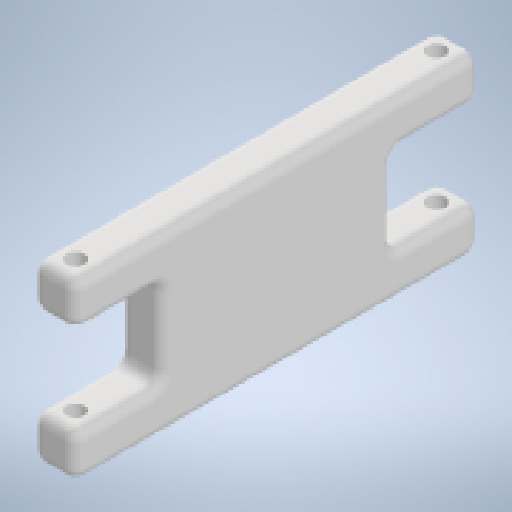
# Autodesk Inventor part: swing pusher
Saved by Autodesk Inventor 2023 (Build 270158000, 158)
## iProperties
Created: 2023-01-25
Part Number: swing pusher
Material: Generic
Document SubType Name: Modeling
Designer: Gabriel - T3 CAD
Density: 1 g/cm^3
Appearance: Default
Mass: 40.324 g
Surface Area: 106.324 cm^2
Volume: 40.324 cm^3
Author: Gabriel - T3 CAD
Autodesk Inventor part; units mm, degrees
ref_plane "YZ Plane" through (0, 0, 0) normal (1, 0, 0) x (0, 1, 0)
ref_plane "XZ Plane" through (0, 0, 0) normal (0, 1, 0) x (-1, 0, 0)
ref_plane "XY Plane" through (0, 0, 0) normal (0, 0, 1) x (1, 0, 0)
sketch "Sketch1" plane through (0, 0, 0) normal (0, 1, 0) x (-1, 0, 0)
  line L0 (0, 0) -> (12.7, 0)
  line L1 (12.7, 0) -> (12.7, 109.3393)
  line L2 (12.7, 109.3393) -> (0, 109.3393)
  line L3 (0, 109.3393) -> (0, 0)
  circle A0 centre (6.35, 6.35) radius 2.5797
  circle A1 centre (6.35, 102.9893) radius 2.5797
  circle A2 centre (6.35, 6.35) radius 6.35
  circle A3 centre (6.35, 102.9893) radius 6.35
  point P0 (0, 102.9893)
  point P1 (0, 6.35)
  point P2 (12.7, 6.35)
  point P3 (12.7, 102.9893)
  dimension "d0" = 12.7
  dimension "d1" = 109.3393
  dimension "d2" = 6.35
  dimension "d3" = 6.35
  dimension "d4" = 5.1594
  dimension "d5" = 6.35
  dimension "d6" = 5.1594
  dimension "d7" = 6.35
  constraints: 8 end point, 4 centre point, 2 coincident, 2 parallel, 1 horizontal, 1 perpendicular
  measures "d0" distance of L2.end L1.end
  measures "d1" distance of L1.end L0.end
  measures "d2" distance from line of L0 A0.centre
  measures "d3" distance from line of L1 A0.centre
  measures "d4" diameter of A0
  measures "d5" distance from line of L1 A1.centre
  measures "d6" diameter of A1
  measures "d7" distance from line of L2 A1.centre
extrude "Extrusion1" add sketch "Sketch1" along normal blind 50.8 contours A2 | L3 A3 L1 A2 | A3
sketch "Sketch5" plane through (0, 0, 102.9893) normal (1, 0, 0) x (0, 0, -1)
  line L0 (102.9893, 0) -> (96.6393, 0) projected
  line L1 (102.9893, 0) -> (-6.35, 0)
  line L2 (-6.35, 0) -> (-6.35, 50.8)
  line L3 (-6.35, 50.8) -> (102.9893, 50.8)
  line L4 (102.9893, 50.8) -> (102.9893, 0)
  line L5 (0, 50.8) -> (96.6393, 50.8) projected
  line L6 (-6.35, 0) -> (-6.35, 50.8) projected
  line L7 (-6.35, 38.1) -> (19.05, 38.1)
  line L8 (19.05, 38.1) -> (19.05, 12.7)
  line L9 (19.05, 12.7) -> (-6.35, 12.7)
  line L10 (-6.35, 12.7) -> (-6.35, 38.1)
  line L11 (102.9893, 0) -> (102.9893, 50.8) projected
  line L12 (102.9893, 38.1) -> (77.5893, 38.1)
  line L13 (77.5893, 38.1) -> (77.5893, 12.7)
  line L14 (77.5893, 12.7) -> (102.9893, 12.7)
  line L15 (102.9893, 12.7) -> (102.9893, 38.1)
  point P0 (6.35, 38.1)
  point P1 (102.9893, 38.1)
  point P2 (-6.35, 38.1)
  point P3 (-6.35, 12.7)
  dimension "d40" = 109.3393
  dimension "d41" = 25.4
  dimension "d42" = 25.4
  dimension "d43" = 12.7
  constraints: 24 end point, 6 parallel, 3 horizontal, 3 perpendicular, 2 collinear, 2 equal length, 2 point on line, 1 midpoint
  measures "d40" distance of L2.end L3.end
  measures "d41" distance of L7.end L8.end
  measures "d42" distance of L7.start L7.end
  measures "d43" distance from line of L5 point (6.35, 38.1)
extrude "Extrusion5" cut sketch "Sketch5" against normal through all contours L14 L13 L12 L4 | L2 L7 L8 L9
fillet "Fillet3" radius 3.175 28 edges at (-6.35, 12.7, 0) (-12.7, 12.7, 15.875) (0, 12.7, 15.875) (-12.7, 0, 54.6697) (-6.35, 0, 109.3393) (0, 0, 54.6697) (-6.35, 0, 0) (-12.7, 50.8, 54.6697) (-6.35, 50.8, 109.3393) (0, 50.8, 54.6697) (-6.35, 50.8, 0) (-6.35, 38.1, 0) (0, 38.1, 15.875) (-12.7, 38.1, 15.875) (-6.35, 12.7, 25.4) (0, 25.4, 25.4) (-12.7, 25.4, 25.4) (-6.35, 38.1, 25.4) (-6.35, 38.1, 109.3393) (-12.7, 38.1, 93.4643) (0, 38.1, 93.4643) (-6.35, 12.7, 109.3393) (-12.7, 12.7, 93.4643) (0, 12.7, 93.4643) (-6.35, 12.7, 83.9393) (0, 25.4, 83.9393) (-12.7, 25.4, 83.9393) (-6.35, 38.1, 83.9393)
body "Solid1"
